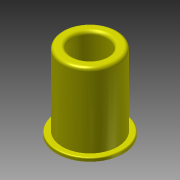
# Autodesk Inventor part: Adaptador rollo 5cm
Saved by Autodesk Inventor 2014 (Build 180170000, 170)
## iProperties
Created: 2017-02-06
Part Number: Adaptador rollo 5cm
Material: Generic
Document SubType Name: Modeling
Designer: Rubén
Density: 1 g/cm^3
Appearance: Smooth - Yellow
Author: Rubén
Autodesk Inventor part; units mm, degrees
ref_plane "YZ Plane" through (0, 0, 0) normal (1, 0, 0) x (0, 1, 0)
ref_plane "XZ Plane" through (0, 0, 0) normal (0, 1, 0) x (-1, 0, 0)
ref_plane "XY Plane" through (0, 0, 0) normal (0, 0, 1) x (1, 0, 0)
sketch "Sketch1" plane through (0, 0, 0) normal (0, 1, 0) x (-1, 0, 0)
  circle A0 centre (0, 0) radius 15.75
  circle A1 centre (0, 0) radius 25
  dimension "d0" = 31.5
  dimension "d1" = 50
  constraints: 2 centre point, 2 coincident
  measures "d0" diameter of A0
  measures "d1" diameter of A1
extrude "Extrusion1" add sketch "Sketch1" along normal blind 70
sketch "Sketch2" plane through (0, 0, 0) normal (0, -1, 0) x (1, 0, 0)
  circle A0 centre (0, 0) radius 25 projected
  circle A1 centre (0, 0) radius 30
  dimension "d4" = 5
  constraints: 1 centre point, 1 coincident
  measures "d4" radial gap between concentric circles of A1 A0
extrude "Extrusion2" add sketch "Sketch2" against normal blind 3
fillet "Fillet1" radius 1 1 edges at (-30, 3, 0)
fillet "Fillet2" radius 3 2 edges at (15.75, 70, 0) (25, 70, 0)
body "Solid1"
